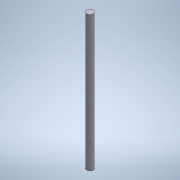
# Autodesk Inventor part: Tij
Saved by Autodesk Inventor 2020 (Build 240168000, 168)
## iProperties
Created: 2021-12-24
Part Number: Tij
Material: Stainless Steel AISI 440C, Welded
Document SubType Name: Modeling
Designer: Umur Batuhan Özmen
Density: 7.8 g/cm^3
Appearance: Weld - Stainless Steel
Author: Umur Batuhan Özmen
Autodesk Inventor part; units mm, degrees
ref_plane "YZ Plane" through (0, 0, 0) normal (1, 0, 0) x (0, 1, 0)
ref_plane "XZ Plane" through (0, 0, 0) normal (0, 1, 0) x (-1, 0, 0)
ref_plane "XY Plane" through (0, 0, 0) normal (0, 0, 1) x (1, 0, 0)
sketch "Sketch1" plane through (0, 0, 0) normal (0, 1, 0) x (-1, 0, 0)
  circle A0 centre (0, 0) radius 4.5
  dimension "d0" = 9
  constraints: 1 centre point, 1 coincident
  measures "d0" diameter of A0
extrude "Extrusion1" add sketch "Sketch1" along normal blind 180
thread "Thread1" size "M9x1.25" class "6g" standard "ANSI Metric M Profile" full length
body "Solid1"
